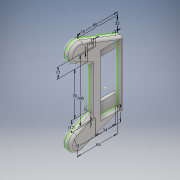
# Autodesk Inventor part: controller
Saved by Autodesk Inventor 2018.3 (Build 223284000, 284)
## iProperties
Created: 2019-10-24
Part Number: controller
Material: 一般
Document SubType Name: Modeling
Designer: Eiji Nishizawa
Density: 1 g/cm^3
Appearance: 既定
Author: Eiji Nishizawa
Autodesk Inventor part; units mm, degrees
ref_plane "YZ Plane" through (0, 0, 0) normal (1, 0, 0) x (0, 1, 0)
ref_plane "XZ Plane" through (0, 0, 0) normal (0, 1, 0) x (-1, 0, 0)
ref_plane "XY Plane" through (0, 0, 0) normal (0, 0, 1) x (1, 0, 0)
sketch "スケッチ1" plane through (0, 0, 0) normal (1, 0, 0) x (0, 1, 0)
  line L0 (17.3083, 65.7844) -> (-16.6917, 65.7844)
  line L1 (-16.6917, 65.7844) -> (-16.6917, -34.2156)
  line L2 (-16.6917, -34.2156) -> (17.3083, -34.2156)
  line L3 (17.3083, -34.2156) -> (17.3083, 65.7844)
  line L4 (19.3083, -36.2156) -> (-18.6917, -36.2156)
  line L5 (-18.6917, -36.2156) -> (-18.6917, 67.7844)
  line L6 (-18.6917, 67.7844) -> (19.3083, 67.7844)
  line L7 (19.3083, 67.7844) -> (19.3083, -36.2156)
  line L8 (19.3083, 67.7844) -> (-45.6917, 92.7844)
  line L9 (19.3083, -36.2156) -> (-45.6917, -61.2156)
  arc A0 (-45.6917, 92.7844) -> (-56.4726, 64.7884) centre (-51.0764, 78.7842) ccw
  arc A1 (-56.8602, -33.3753) -> (-45.6917, -61.2156) centre (-51.0764, -47.2154) ccw
  line L10 (-56.4726, 64.7884) -> (-28.6917, 50.7844)
  line L11 (-28.6917, 50.7844) -> (-28.6917, -19.2156)
  line L12 (-28.6917, -19.2156) -> (-56.8602, -33.3753)
  point P0 (0, 0)
  dimension "d0" = 34
  dimension "d1" = 100
  dimension "d2" = 2
  dimension "d3" = 2
  dimension "d4" = 2
  dimension "d5" = 2
  dimension "d6" = 15
  dimension "d7" = 15
  dimension "d8" = 25
  dimension "d9" = 65
  dimension "d10" = 25
  dimension "d11" = 65
  dimension "d12" = 70
  dimension "d13" = 17
  dimension "d14" = 17
  dimension "d15" = 10
  constraints: 26 end point, 4 parallel, 4 point on circle, 2 centre point, 2 horizontal, 2 perpendicular, 2 tangent, 1 vertical
  measures "d0" distance of L1.end L2.end
  measures "d1" distance between parallel lines of L2 L0
  measures "d2" distance between parallel lines of L6 L0
  measures "d3" distance between parallel lines of L5 L1
  measures "d4" distance between parallel lines of L4 L2
  measures "d5" distance between parallel lines of L3 L7
  measures "d6" radius of A1
  measures "d7" radius of A0
  measures "d8" vertical distance of L6.end L8.end
  measures "d9" horizontal distance of L6.end L8.end
  measures "d10" vertical distance of L4.start L9.end
  measures "d11" horizontal distance of L4.start L9.end
  measures "d12" distance of L10.end L11.end
  measures "d13" distance from line of L10.end L6
  measures "d14" vertical distance of L11.end L4.end
  measures "d15" distance between parallel lines of L5 L11
extrude "押し出し1" add sketch "スケッチ1" against normal blind 5 contours L3 L2 L1 L0 | L9 A1 L12 L11 L10 A0 L8 L6 L5 L4 | L4 L5 L6 L7
extrude "押し出し2" add sketch "スケッチ1" along normal blind 9
fillet "フィレット1" radius 4 6 edges at (9, -65.0744, 84.1746) (9, -13.1917, 80.2844) (9, -42.5822, 57.7864) (9, -42.776, -26.2955) (9, -13.1917, -48.7156) (9, -64.998, -52.8002)
sketch "スケッチ2" plane through (-5, 0, 0) normal (-1, 0, 0) x (0, 0, 1)
  line L0 (-19.2156, -28.6917) -> (50.7844, -28.6917) projected
  line L1 (-16.2156, 19.3083) -> (47.7844, 19.3083)
  line L2 (47.7844, 19.3083) -> (47.7844, -28.6917)
  line L3 (47.7844, -28.6917) -> (-16.2156, -28.6917)
  line L4 (-16.2156, -28.6917) -> (-16.2156, 19.3083)
  line L5 (67.7844, 19.3083) -> (-36.2156, 19.3083) projected
  point P0 (0, 0)
  dimension "d21" = 64
  dimension "d22" = 3
  dimension "d23" = 3
  dimension "d26" = 0
  constraints: 8 end point, 2 parallel, 1 horizontal, 1 perpendicular, 1 point on line
  measures "d21" distance of L1.start L1.end
  measures "d22" distance from line of L0.end L2
  measures "d23" distance from line of L0.start L4
  measures "d26" distance between parallel lines of L5 L1
extrude "押し出し3" cut sketch "スケッチ2" against normal blind 5
fillet "フィレット2" radius 4 6 edges at (-5, -13.1917, 80.2844) (-5, -65.0744, 84.1746) (-5, -13.1917, -48.7156) (-5, -64.998, -52.8002) (-5, -42.776, -26.2955) (-5, -42.5822, 57.7864)
